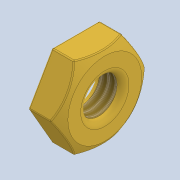
# Autodesk Inventor part: M4_Nut
Saved by Autodesk Inventor 2021.2 (Build 252289000, 289)
## iProperties
Created: 2020-02-10
Part Number: M4_Nut
Material: 鉄、鋳鉄
Document SubType Name: Modeling
Designer: Hagihara Yuya
Density: 7.15 g/cm^3
Appearance: ゴールド
Author: Hagihara Yuya
Autodesk Inventor part; units mm, degrees
ref_plane "YZ Plane" through (0, 0, 0) normal (1, 0, 0) x (0, 1, 0)
ref_plane "XZ Plane" through (0, 0, 0) normal (0, 1, 0) x (-1, 0, 0)
ref_plane "XY Plane" through (0, 0, 0) normal (0, 0, 1) x (1, 0, 0)
sketch "スケッチ1" plane through (0, 0, 0) normal (1, 0, 0) x (0, 1, 0)
  line L0 (0, -3.1754) -> (-2.75, -1.5877)
  line L1 (-2.75, -1.5877) -> (-2.75, 1.5877)
  line L2 (-2.75, 1.5877) -> (0, 3.1754)
  line L3 (0, 3.1754) -> (2.75, 1.5877)
  line L4 (2.75, 1.5877) -> (2.75, -1.5877)
  line L5 (2.75, -1.5877) -> (0, -3.1754)
  line L6 (0, -4.4456) -> (0, 4.4456) projected
  point P0 (0, 0)
  point P1 (0, 0)
  dimension "d0" = 5.5
  constraints: 12 end point, 1 coincident, 1 point on line, 13 other
  measures "d0" distance between parallel lines of L1 L4
extrude "押し出し1" add sketch "スケッチ1" along normal blind 2
sketch "スケッチ2" plane through (2, 0, 0) normal (1, 0, 0) x (0, 0, -1)
  point P0 (0, 0)
  point P1 (0, 0)
  constraints: 1 coincident
hole "穴1" at (2, 0, 0) direction (-1, 0, 0) diameter 2.459 end through all thread size "M3x0.5" class "6H" standard "ISO Metric profile"
sketch "スケッチ5" plane through (0, 0, 0) normal (0, 1, 0) x (-1, 0, 0)
  circle A0 centre (2.126, 0) radius 4.8199
  line L0 (7.8863, 0) -> (-4.853, 0) projected
  line L1 (0, 1.5877) -> (0, 3.1754) projected
  line L2 (0, 3.1754) -> (-2, 3.1754) projected
  line L3 (-2, -1.5877) -> (-2, -3.1754) projected
  circle A1 centre (2.126, 0) radius 5.2065
  point P0 (0, 0)
  point P1 (-1.5, 3.1754)
  point P2 (-1.9, 2.65)
  point P3 (-3.0804, 0)
  point P4 (-2.6939, 0)
  point P5 (6.9459, 0)
  point P6 (7.3325, 0)
  dimension "d14" = 1.5
  dimension "d15" = 2.65
  dimension "d16" = 1.9
  constraints: 2 point on circle, 2 point on line, 1 centre point, 1 coincident, 3 other
  measures "d14" distance of L1.end A0.start
  measures "d15" distance from line of L0 A0.end
  measures "d16" distance from line of L1 A0.end
revolve "回転1" cut sketch "スケッチ5" angle 360 about axis through (-10, 0, 0) along (1, 0, 0) contours A0 L2 A1 L0 | A0 L0 A1 L2
fillet "フィレット1" radius 0.1 12 edges at (0.75, 0, 3.1754) (0.75, -2.75, 1.5877) (0.75, -2.75, -1.5877) (0.75, 0, -3.1754) (0.75, 2.75, -1.5877) (0.75, 2.75, 1.5877) (0, 2.75, 0) (0, 1.375, 2.3816) (0, 1.375, -2.3816) (0, -1.375, -2.3816) (0, -2.75, 0) (0, -1.375, 2.3816)
fillet "フィレット2" radius 0.4 2 edges at (2, 0, 1.2295) (0, 0, 1.2295)
fillet "フィレット3" radius 0.1 13 edges at (1.5164, -0.0259, 3.1565) (1.5135, -2.7366, 1.58) (1.5135, 2.7366, 1.58) (1.5164, 0.0259, 3.1565) (1.8324, 1.375, 2.3816) (1.8324, 2.75, 0) (1.5135, 2.7366, -1.58) (1.8324, 1.375, -2.3816) (1.5135, 0, -3.16) (1.8324, -1.375, -2.3816) (1.5135, -2.7366, -1.58) (1.8324, -2.75, 0) (1.8324, -1.375, 2.3816)
